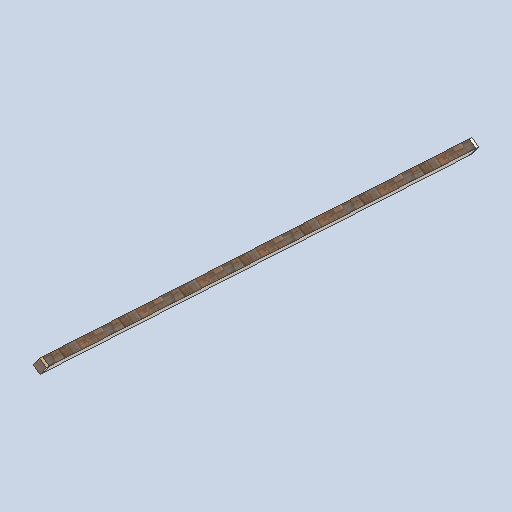
# Autodesk Inventor part: support_beam_segment_0104
Saved by Autodesk Inventor 2024.2 (Build 282272000, 272)
## iProperties
Created: 2024-05-20
Part Number: support_beam_segment_0104
Material: Wood Shake
Document SubType Name: Modeling
Designer: LOSTER_1
Density: 0.4 g/cm^3
Appearance: Shake - Handsplit
Author: LOSTER_1
Autodesk Inventor part; units mm, degrees
ref_plane "YZ Plane" through (0, 0, 0) normal (1, 0, 0) x (0, 1, 0)
ref_plane "XZ Plane" through (0, 0, 0) normal (0, 1, 0) x (-1, 0, 0)
sketch "Sketch1" plane through (0, 0, 0) normal (0, 0, 1) x (1, 0, 0)
  line L0 (-106.7972, -199.4212) -> (-221.5168, -363.2486)
  line L1 (16.0733, -285.461) -> (-106.7972, -199.4212)
  line L2 (16.6111, -285.8734) -> (-98.1042, -449.7038)
  line L3 (-98.1042, -449.7038) -> (-220.977, -363.6673)
  line L4 (-97.5688, -450.1195) -> (17.1869, -286.2407)
  line L5 (17.1869, -286.2407) -> (-106.7972, -199.4212)
  line L6 (-106.7972, -199.4212) -> (-221.5529, -363.3)
  line L7 (-221.5529, -363.3) -> (-97.5688, -450.1195)
  line L8 (-97.5688, -450.1195) -> (-106.7972, -199.4212) construction
  line L9 (17.1869, -286.2407) -> (-221.5529, -363.3) construction
  point P0 (0, 0)
  point P1 (-102.183, -324.7704)
  constraints: 20 end point, 2 midpoint, 2 parallel, 2 perpendicular
ref_plane "Work Plane2" through (0, 0, 7900) normal (0, 0, 1) x (1, 0, 0)
ref_plane "Work Plane1" through (0, 0, 0) normal (0, 0, 1) x (1, 0, 0)
sketch "Sketch2" plane through (0, 0, 7900) normal (0, 0, 1) x (1, 0, 0)
  line L0 (214.7789, 359.5081) -> (91.9061, 445.5446) construction
  line L1 (91.9061, 445.5446) -> (-22.8092, 281.7142) construction
  line L2 (100.0636, 195.6777) -> (214.7789, 359.5081) construction
  line L3 (-22.8092, 281.7142) -> (100.0636, 195.6777) construction
  line L4 (100.0636, 195.6777) -> (214.7789, 359.5081)
  line L5 (214.7789, 359.5081) -> (91.9061, 445.5446)
  line L6 (91.9061, 445.5446) -> (-22.8092, 281.7142)
  line L7 (-22.8092, 281.7142) -> (100.0636, 195.6777)
  line L8 (100.0636, 195.6777) -> (91.9061, 445.5446) construction
  line L9 (214.7789, 359.5081) -> (-22.8092, 281.7142) construction
  point P0 (0, 0)
  point P1 (95.9849, 320.6112)
  constraints: 12 end point, 2 midpoint, 2 parallel, 1 perpendicular
loft "Loft1" add profiles "Sketch1", "Sketch2"
sketch "Sketch3" plane through (-97.5688, -450.1195, 0) normal (0, 0, -1) x (-0.8191, 0.5736, 0)
  line L0 (0, 0) -> (0, 200.0628) projected
  line L1 (151.3594, 0) -> (0, 0) projected
  line L2 (151.3594, 200.0628) -> (151.3594, 0) projected
  line L3 (0, 200.0628) -> (151.3594, 200.0628) projected
  point P0 (178.2656, 424.6747)
sketch "Sketch4" plane through (100.0636, 195.6777, 7900) normal (0, 0, 1) x (0.8192, -0.5736, 0)
  line L0 (0, 0) -> (0, 200) projected
  line L1 (0, 200) -> (-150, 200) projected
  line L2 (-150, 200) -> (-150, 0) projected
  line L3 (-150, 0) -> (0, 0) projected
  point P0 (30.2688, -217.684)
extrude "Extrusion1" add sketch "Sketch3" along normal blind 50
extrude "Extrusion2" add sketch "Sketch4" along normal blind 50
body "Solid1"
